Autodesk Fusion 360 part; units mm, degrees
(part 3 of 3)
sketch "Sketch2" plane through (0, 0, 6.5) normal (0, 0, 1) x (-1, 0, 0)
  line L0 (9.947362, -2.78719) -> (10.269334, 2.51736)
  arc A0 (9.726793, 3.184436) -> (10.269334, 2.51736) centre (10.86723, 3.557802) ccw
  arc A1 (9.726793, 3.184436) -> (9.129617, 4.626145) centre (0, 0) ccw
  arc A2 (9.548298, 6.176136) -> (9.129617, 4.626145) centre (10.200038, 5.168547) ccw
  line L1 (9.548298, 6.176136) -> (11.361886, 7.34922)
  spline S0 degree 5 poles (11.361886, 7.34922) (11.373267, 7.356582) (11.395716, 7.371712) (11.42845, 7.395628) (11.470315, 7.429836) (11.52024, 7.475743) (11.568461, 7.523898) (11.615662, 7.57342) (11.662318, 7.623687) (11.708575, 7.674485) (11.754381, 7.725854) (11.799563, 7.777982) (11.843926, 7.831092) (11.887356, 7.885306) (11.929863, 7.940601) (11.971521, 7.996873) (12.012444, 8.053973) (12.052738, 8.111759) (12.092468, 8.170145) (12.131644, 8.229106) (12.170248, 8.288657) (12.208248, 8.348827) (12.245612, 8.409646) (12.28233, 8.471119) (12.318409, 8.533228) (12.353869, 8.595944) (12.388733, 8.659229) (12.423021, 8.723051) (12.456745, 8.78739) (12.489908, 8.852234) (12.522508, 8.917579) (12.554541, 8.983424) (12.586002, 9.049766) (12.616893, 9.1166) (12.647217, 9.183915) (12.676977, 9.251698) (12.706181, 9.319937) (12.734832, 9.38862) (12.762935, 9.457736) (12.790491, 9.527279) (12.8175, 9.597241) (12.843962, 9.667617) (12.869878, 9.738401) (12.895248, 9.809586) (12.920074, 9.881166) (12.944358, 9.953133) (12.968101, 10.025479) (12.991304, 10.098198) (13.013969, 10.171282) (13.036098, 10.244727) (13.057689, 10.318525) (13.078745, 10.392671) (13.099265, 10.46716) (13.119249, 10.541987) (13.1387, 10.617144) (13.157616, 10.692627) (13.176, 10.768429) (13.19385, 10.844546) (13.211169, 10.920971) (13.227957, 10.997702) (13.244213, 11.074732) (13.259939, 11.152056) (13.275135, 11.229671) (13.289801, 11.307571) (13.303937, 11.385749) (13.317543, 11.464201) (13.33062, 11.54292) (13.343167, 11.621902) (13.355185, 11.701142) (13.366676, 11.780639) (13.377639, 11.860389) (13.385988, 11.924391) (13.392014, 11.972507) (13.395926, 12.004634) (13.397855, 12.02071) knots 0 0 0 0 0 0 0.01428571 0.02857143 0.04285714 0.05714286 0.07142857 0.08571429 0.1 0.11428571 0.12857143 0.14285714 0.15714286 0.17142857 0.18571429 0.2 0.21428571 0.22857143 0.24285714 0.25714286 0.27142857 0.28571429 0.3 0.31428571 0.32857143 0.34285714 0.35714286 0.37142857 0.38571429 0.4 0.41428571 0.42857143 0.44285714 0.45714286 0.47142857 0.48571429 0.5 0.51428571 0.52857143 0.54285714 0.55714286 0.57142857 0.58571429 0.6 0.61428571 0.62857143 0.64285714 0.65714286 0.67142857 0.68571429 0.7 0.71428571 0.72857143 0.74285714 0.75714286 0.77142857 0.78571429 0.8 0.81428571 0.82857143 0.84285714 0.85714286 0.87142857 0.88571429 0.9 0.91428571 0.92857143 0.94285714 0.95714286 0.97142857 0.98571429 1 1 1 1 1 1
  arc A3 (13.397855, 12.02071) -> (12.02071, 13.397855) centre (0, 0) ccw
  spline S1 degree 5 poles (12.02071, 13.397855) (12.004634, 13.395926) (11.972507, 13.392014) (11.924391, 13.385988) (11.860389, 13.377639) (11.780639, 13.366676) (11.701142, 13.355185) (11.621902, 13.343167) (11.54292, 13.33062) (11.464201, 13.317543) (11.385749, 13.303937) (11.307571, 13.289801) (11.229671, 13.275135) (11.152056, 13.259939) (11.074732, 13.244213) (10.997702, 13.227957) (10.920971, 13.211169) (10.844546, 13.19385) (10.768429, 13.176) (10.692627, 13.157616) (10.617144, 13.1387) (10.541987, 13.119249) (10.46716, 13.099265) (10.392671, 13.078745) (10.318525, 13.057689) (10.244727, 13.036098) (10.171282, 13.013969) (10.098198, 12.991304) (10.025479, 12.968101) (9.953133, 12.944358) (9.881166, 12.920074) (9.809586, 12.895248) (9.738401, 12.869878) (9.667617, 12.843962) (9.597241, 12.8175) (9.527279, 12.790491) (9.457736, 12.762935) (9.38862, 12.734832) (9.319937, 12.706181) (9.251698, 12.676977) (9.183915, 12.647217) (9.1166, 12.616893) (9.049766, 12.586002) (8.983424, 12.554541) (8.917579, 12.522508) (8.852234, 12.489908) (8.78739, 12.456745) (8.723051, 12.423021) (8.659229, 12.388733) (8.595944, 12.353869) (8.533228, 12.318409) (8.471119, 12.28233) (8.409646, 12.245612) (8.348827, 12.208248) (8.288657, 12.170248) (8.229106, 12.131644) (8.170145, 12.092468) (8.111759, 12.052738) (8.053973, 12.012444) (7.996873, 11.971521) (7.940601, 11.929863) (7.885306, 11.887356) (7.831092, 11.843926) (7.777982, 11.799563) (7.725854, 11.754381) (7.674485, 11.708575) (7.623687, 11.662318) (7.57342, 11.615662) (7.523898, 11.568461) (7.475743, 11.52024) (7.429836, 11.470315) (7.395628, 11.42845) (7.371712, 11.395716) (7.356582, 11.373267) (7.34922, 11.361886) knots -1 -1 -1 -1 -1 -1 -0.98571429 -0.97142857 -0.95714286 -0.94285714 -0.92857143 -0.91428571 -0.9 -0.88571429 -0.87142857 -0.85714286 -0.84285714 -0.82857143 -0.81428571 -0.8 -0.78571429 -0.77142857 -0.75714286 -0.74285714 -0.72857143 -0.71428571 -0.7 -0.68571429 -0.67142857 -0.65714286 -0.64285714 -0.62857143 -0.61428571 -0.6 -0.58571429 -0.57142857 -0.55714286 -0.54285714 -0.52857143 -0.51428571 -0.5 -0.48571429 -0.47142857 -0.45714286 -0.44285714 -0.42857143 -0.41428571 -0.4 -0.38571429 -0.37142857 -0.35714286 -0.34285714 -0.32857143 -0.31428571 -0.3 -0.28571429 -0.27142857 -0.25714286 -0.24285714 -0.22857143 -0.21428571 -0.2 -0.18571429 -0.17142857 -0.15714286 -0.14285714 -0.12857143 -0.11428571 -0.1 -0.08571429 -0.07142857 -0.05714286 -0.04285714 -0.02857143 -0.01428571 0 0 0 0 0 0
  line L2 (7.34922, 11.361886) -> (6.176136, 9.548298)
  arc A4 (4.626145, 9.129617) -> (6.176136, 9.548298) centre (5.168547, 10.200038) ccw
  arc A5 (4.626145, 9.129617) -> (3.184436, 9.726793) centre (0, 0) ccw
  arc A6 (3.025234, 9.791883) -> (3.184436, 9.726793) centre (3.557802, 10.86723) ccw
  line L3 (3.025234, 9.791883) -> (-3.025234, 9.791883)
  arc A7 (-3.184436, 9.726793) -> (-3.025234, 9.791883) centre (-3.557802, 10.86723) ccw
  arc A8 (-3.184436, 9.726793) -> (-4.626145, 9.129617) centre (0, 0) ccw
  arc A9 (-6.176136, 9.548298) -> (-4.626145, 9.129617) centre (-5.168547, 10.200038) ccw
  line L4 (-6.176136, 9.548298) -> (-7.34922, 11.361886)
  spline S2 degree 5 poles (-7.34922, 11.361886) (-7.356582, 11.373267) (-7.371712, 11.395716) (-7.395628, 11.42845) (-7.429836, 11.470315) (-7.475743, 11.52024) (-7.523898, 11.568461) (-7.57342, 11.615662) (-7.623687, 11.662318) (-7.674485, 11.708575) (-7.725854, 11.754381) (-7.777982, 11.799563) (-7.831092, 11.843926) (-7.885306, 11.887356) (-7.940601, 11.929863) (-7.996873, 11.971521) (-8.053973, 12.012444) (-8.111759, 12.052738) (-8.170145, 12.092468) (-8.229106, 12.131644) (-8.288657, 12.170248) (-8.348827, 12.208248) (-8.409646, 12.245612) (-8.471119, 12.28233) (-8.533228, 12.318409) (-8.595944, 12.353869) (-8.659229, 12.388733) (-8.723051, 12.423021) (-8.78739, 12.456745) (-8.852234, 12.489908) (-8.917579, 12.522508) (-8.983424, 12.554541) (-9.049766, 12.586002) (-9.1166, 12.616893) (-9.183915, 12.647217) (-9.251698, 12.676977) (-9.319937, 12.706181) (-9.38862, 12.734832) (-9.457736, 12.762935) (-9.527279, 12.790491) (-9.597241, 12.8175) (-9.667617, 12.843962) (-9.738401, 12.869878) (-9.809586, 12.895248) (-9.881166, 12.920074) (-9.953133, 12.944358) (-10.025479, 12.968101) (-10.098198, 12.991304) (-10.171282, 13.013969) (-10.244727, 13.036098) (-10.318525, 13.057689) (-10.392671, 13.078745) (-10.46716, 13.099265) (-10.541987, 13.119249) (-10.617144, 13.1387) (-10.692627, 13.157616) (-10.768429, 13.176) (-10.844546, 13.19385) (-10.920971, 13.211169) (-10.997702, 13.227957) (-11.074732, 13.244213) (-11.152056, 13.259939) (-11.229671, 13.275135) (-11.307571, 13.289801) (-11.385749, 13.303937) (-11.464201, 13.317543) (-11.54292, 13.33062) (-11.621902, 13.343167) (-11.701142, 13.355185) (-11.780639, 13.366676) (-11.860389, 13.377639) (-11.924391, 13.385988) (-11.972507, 13.392014) (-12.004634, 13.395926) (-12.02071, 13.397855) knots 0 0 0 0 0 0 0.01428571 0.02857143 0.04285714 0.05714286 0.07142857 0.08571429 0.1 0.11428571 0.12857143 0.14285714 0.15714286 0.17142857 0.18571429 0.2 0.21428571 0.22857143 0.24285714 0.25714286 0.27142857 0.28571429 0.3 0.31428571 0.32857143 0.34285714 0.35714286 0.37142857 0.38571429 0.4 0.41428571 0.42857143 0.44285714 0.45714286 0.47142857 0.48571429 0.5 0.51428571 0.52857143 0.54285714 0.55714286 0.57142857 0.58571429 0.6 0.61428571 0.62857143 0.64285714 0.65714286 0.67142857 0.68571429 0.7 0.71428571 0.72857143 0.74285714 0.75714286 0.77142857 0.78571429 0.8 0.81428571 0.82857143 0.84285714 0.85714286 0.87142857 0.88571429 0.9 0.91428571 0.92857143 0.94285714 0.95714286 0.97142857 0.98571429 1 1 1 1 1 1
  arc A10 (-12.02071, 13.397855) -> (-13.397855, 12.02071) centre (0, 0) ccw
  spline S3 degree 5 poles (-13.397855, 12.02071) (-13.395926, 12.004634) (-13.392014, 11.972507) (-13.385988, 11.924391) (-13.377639, 11.860389) (-13.366676, 11.780639) (-13.355185, 11.701142) (-13.343167, 11.621902) (-13.33062, 11.54292) (-13.317543, 11.464201) (-13.303937, 11.385749) (-13.289801, 11.307571) (-13.275135, 11.229671) (-13.259939, 11.152056) (-13.244213, 11.074732) (-13.227957, 10.997702) (-13.211169, 10.920971) (-13.19385, 10.844546) (-13.176, 10.768429) (-13.157616, 10.692627) (-13.1387, 10.617144) (-13.119249, 10.541987) (-13.099265, 10.46716) (-13.078745, 10.392671) (-13.057689, 10.318525) (-13.036098, 10.244727) (-13.013969, 10.171282) (-12.991304, 10.098198) (-12.968101, 10.025479) (-12.944358, 9.953133) (-12.920074, 9.881166) (-12.895248, 9.809586) (-12.869878, 9.738401) (-12.843962, 9.667617) (-12.8175, 9.597241) (-12.790491, 9.527279) (-12.762935, 9.457736) (-12.734832, 9.38862) (-12.706181, 9.319937) (-12.676977, 9.251698) (-12.647217, 9.183915) (-12.616893, 9.1166) (-12.586002, 9.049766) (-12.554541, 8.983424) (-12.522508, 8.917579) (-12.489908, 8.852234) (-12.456745, 8.78739) (-12.423021, 8.723051) (-12.388733, 8.659229) (-12.353869, 8.595944) (-12.318409, 8.533228) (-12.28233, 8.471119) (-12.245612, 8.409646) (-12.208248, 8.348827) (-12.170248, 8.288657) (-12.131644, 8.229106) (-12.092468, 8.170145) (-12.052738, 8.111759) (-12.012444, 8.053973) (-11.971521, 7.996873) (-11.929863, 7.940601) (-11.887356, 7.885306) (-11.843926, 7.831092) (-11.799563, 7.777982) (-11.754381, 7.725854) (-11.708575, 7.674485) (-11.662318, 7.623687) (-11.615662, 7.57342) (-11.568461, 7.523898) (-11.52024, 7.475743) (-11.470315, 7.429836) (-11.42845, 7.395628) (-11.395716, 7.371712) (-11.373267, 7.356582) (-11.361886, 7.34922) knots -1 -1 -1 -1 -1 -1 -0.98571429 -0.97142857 -0.95714286 -0.94285714 -0.92857143 -0.91428571 -0.9 -0.88571429 -0.87142857 -0.85714286 -0.84285714 -0.82857143 -0.81428571 -0.8 -0.78571429 -0.77142857 -0.75714286 -0.74285714 -0.72857143 -0.71428571 -0.7 -0.68571429 -0.67142857 -0.65714286 -0.64285714 -0.62857143 -0.61428571 -0.6 -0.58571429 -0.57142857 -0.55714286 -0.54285714 -0.52857143 -0.51428571 -0.5 -0.48571429 -0.47142857 -0.45714286 -0.44285714 -0.42857143 -0.41428571 -0.4 -0.38571429 -0.37142857 -0.35714286 -0.34285714 -0.32857143 -0.31428571 -0.3 -0.28571429 -0.27142857 -0.25714286 -0.24285714 -0.22857143 -0.21428571 -0.2 -0.18571429 -0.17142857 -0.15714286 -0.14285714 -0.12857143 -0.11428571 -0.1 -0.08571429 -0.07142857 -0.05714286 -0.04285714 -0.02857143 -0.01428571 0 0 0 0 0 0
  line L5 (-11.361886, 7.34922) -> (-9.548298, 6.176136)
  arc A11 (-9.129617, 4.626145) -> (-9.548298, 6.176136) centre (-10.200038, 5.168547) ccw
  arc A12 (-9.129617, 4.626145) -> (-9.726793, 3.184436) centre (0, 0) ccw
  arc A13 (-10.545247, 2.401806) -> (-9.726793, 3.184436) centre (-10.86723, 3.557802) ccw
  line L6 (-10.545247, 2.401806) -> (-9.854685, -2.913789)
  arc A14 (-9.726793, -3.184436) -> (-9.854685, -2.913789) centre (-10.86723, -3.557802) ccw
  arc A15 (-9.726793, -3.184436) -> (-9.129617, -4.626145) centre (0, 0) ccw
  arc A16 (-9.548298, -6.176136) -> (-9.129617, -4.626145) centre (-10.200038, -5.168547) ccw
  line L7 (-9.548298, -6.176136) -> (-11.361886, -7.34922)
  spline S4 degree 5 poles (-11.361886, -7.34922) (-11.373267, -7.356582) (-11.395716, -7.371712) (-11.42845, -7.395628) (-11.470315, -7.429836) (-11.52024, -7.475743) (-11.568461, -7.523898) (-11.615662, -7.57342) (-11.662318, -7.623687) (-11.708575, -7.674485) (-11.754381, -7.725854) (-11.799563, -7.777982) (-11.843926, -7.831092) (-11.887356, -7.885306) (-11.929863, -7.940601) (-11.971521, -7.996873) (-12.012444, -8.053973) (-12.052738, -8.111759) (-12.092468, -8.170145) (-12.131644, -8.229106) (-12.170248, -8.288657) (-12.208248, -8.348827) (-12.245612, -8.409646) (-12.28233, -8.471119) (-12.318409, -8.533228) (-12.353869, -8.595944) (-12.388733, -8.659229) (-12.423021, -8.723051) (-12.456745, -8.78739) (-12.489908, -8.852234) (-12.522508, -8.917579) (-12.554541, -8.983424) (-12.586002, -9.049766) (-12.616893, -9.1166) (-12.647217, -9.183915) (-12.676977, -9.251698) (-12.706181, -9.319937) (-12.734832, -9.38862) (-12.762935, -9.457736) (-12.790491, -9.527279) (-12.8175, -9.597241) (-12.843962, -9.667617) (-12.869878, -9.738401) (-12.895248, -9.809586) (-12.920074, -9.881166) (-12.944358, -9.953133) (-12.968101, -10.025479) (-12.991304, -10.098198) (-13.013969, -10.171282) (-13.036098, -10.244727) (-13.057689, -10.318525) (-13.078745, -10.392671) (-13.099265, -10.46716) (-13.119249, -10.541987) (-13.1387, -10.617144) (-13.157616, -10.692627) (-13.176, -10.768429) (-13.19385, -10.844546) (-13.211169, -10.920971) (-13.227957, -10.997702) (-13.244213, -11.074732) (-13.259939, -11.152056) (-13.275135, -11.229671) (-13.289801, -11.307571) (-13.303937, -11.385749) (-13.317543, -11.464201) (-13.33062, -11.54292) (-13.343167, -11.621902) (-13.355185, -11.701142) (-13.366676, -11.780639) (-13.377639, -11.860389) (-13.385988, -11.924391) (-13.392014, -11.972507) (-13.395926, -12.004634) (-13.397855, -12.02071) knots 0 0 0 0 0 0 0.01428571 0.02857143 0.04285714 0.05714286 0.07142857 0.08571429 0.1 0.11428571 0.12857143 0.14285714 0.15714286 0.17142857 0.18571429 0.2 0.21428571 0.22857143 0.24285714 0.25714286 0.27142857 0.28571429 0.3 0.31428571 0.32857143 0.34285714 0.35714286 0.37142857 0.38571429 0.4 0.41428571 0.42857143 0.44285714 0.45714286 0.47142857 0.48571429 0.5 0.51428571 0.52857143 0.54285714 0.55714286 0.57142857 0.58571429 0.6 0.61428571 0.62857143 0.64285714 0.65714286 0.67142857 0.68571429 0.7 0.71428571 0.72857143 0.74285714 0.75714286 0.77142857 0.78571429 0.8 0.81428571 0.82857143 0.84285714 0.85714286 0.87142857 0.88571429 0.9 0.91428571 0.92857143 0.94285714 0.95714286 0.97142857 0.98571429 1 1 1 1 1 1
  arc A17 (-13.397855, -12.02071) -> (-12.02071, -13.397855) centre (0, 0) ccw
  spline S5 degree 5 poles (-12.02071, -13.397855) (-12.004634, -13.395926) (-11.972507, -13.392014) (-11.924391, -13.385988) (-11.860389, -13.377639) (-11.780639, -13.366676) (-11.701142, -13.355185) (-11.621902, -13.343167) (-11.54292, -13.33062) (-11.464201, -13.317543) (-11.385749, -13.303937) (-11.307571, -13.289801) (-11.229671, -13.275135) (-11.152056, -13.259939) (-11.074732, -13.244213) (-10.997702, -13.227957) (-10.920971, -13.211169) (-10.844546, -13.19385) (-10.768429, -13.176) (-10.692627, -13.157616) (-10.617144, -13.1387) (-10.541987, -13.119249) (-10.46716, -13.099265) (-10.392671, -13.078745) (-10.318525, -13.057689) (-10.244727, -13.036098) (-10.171282, -13.013969) (-10.098198, -12.991304) (-10.025479, -12.968101) (-9.953133, -12.944358) (-9.881166, -12.920074) (-9.809586, -12.895248) (-9.738401, -12.869878) (-9.667617, -12.843962) (-9.597241, -12.8175) (-9.527279, -12.790491) (-9.457736, -12.762935) (-9.38862, -12.734832) (-9.319937, -12.706181) (-9.251698, -12.676977) (-9.183915, -12.647217) (-9.1166, -12.616893) (-9.049766, -12.586002) (-8.983424, -12.554541) (-8.917579, -12.522508) (-8.852234, -12.489908) (-8.78739, -12.456745) (-8.723051, -12.423021) (-8.659229, -12.388733) (-8.595944, -12.353869) (-8.533228, -12.318409) (-8.471119, -12.28233) (-8.409646, -12.245612) (-8.348827, -12.208248) (-8.288657, -12.170248) (-8.229106, -12.131644) (-8.170145, -12.092468) (-8.111759, -12.052738) (-8.053973, -12.012444) (-7.996873, -11.971521) (-7.940601, -11.929863) (-7.885306, -11.887356) (-7.831092, -11.843926) (-7.777982, -11.799563) (-7.725854, -11.754381) (-7.674485, -11.708575) (-7.623687, -11.662318) (-7.57342, -11.615662) (-7.523898, -11.568461) (-7.475743, -11.52024) (-7.429836, -11.470315) (-7.395628, -11.42845) (-7.371712, -11.395716) (-7.356582, -11.373267) (-7.34922, -11.361886) knots -1 -1 -1 -1 -1 -1 -0.98571429 -0.97142857 -0.95714286 -0.94285714 -0.92857143 -0.91428571 -0.9 -0.88571429 -0.87142857 -0.85714286 -0.84285714 -0.82857143 -0.81428571 -0.8 -0.78571429 -0.77142857 -0.75714286 -0.74285714 -0.72857143 -0.71428571 -0.7 -0.68571429 -0.67142857 -0.65714286 -0.64285714 -0.62857143 -0.61428571 -0.6 -0.58571429 -0.57142857 -0.55714286 -0.54285714 -0.52857143 -0.51428571 -0.5 -0.48571429 -0.47142857 -0.45714286 -0.44285714 -0.42857143 -0.41428571 -0.4 -0.38571429 -0.37142857 -0.35714286 -0.34285714 -0.32857143 -0.31428571 -0.3 -0.28571429 -0.27142857 -0.25714286 -0.24285714 -0.22857143 -0.21428571 -0.2 -0.18571429 -0.17142857 -0.15714286 -0.14285714 -0.12857143 -0.11428571 -0.1 -0.08571429 -0.07142857 -0.05714286 -0.04285714 -0.02857143 -0.01428571 0 0 0 0 0 0
  line L8 (-7.34922, -11.361886) -> (-6.176136, -9.548298)
  arc A18 (-4.626145, -9.129617) -> (-6.176136, -9.548298) centre (-5.168547, -10.200038) ccw
  arc A19 (-4.626145, -9.129617) -> (-3.184436, -9.726793) centre (0, 0) ccw
  arc A20 (-2.770942, -9.961222) -> (-3.184436, -9.726793) centre (-3.557802, -10.86723) ccw
  line L9 (-2.770942, -9.961222) -> (2.770942, -9.961222)
  arc A21 (3.184436, -9.726793) -> (2.770942, -9.961222) centre (3.557802, -10.86723) ccw
  arc A22 (3.184436, -9.726793) -> (4.626145, -9.129617) centre (0, 0) ccw
  arc A23 (6.176136, -9.548298) -> (4.626145, -9.129617) centre (5.168547, -10.200038) ccw
  line L10 (6.176136, -9.548298) -> (7.34922, -11.361886)
  spline S6 degree 5 poles (7.34922, -11.361886) (7.356582, -11.373267) (7.371712, -11.395716) (7.395628, -11.42845) (7.429836, -11.470315) (7.475743, -11.52024) (7.523898, -11.568461) (7.57342, -11.615662) (7.623687, -11.662318) (7.674485, -11.708575) (7.725854, -11.754381) (7.777982, -11.799563) (7.831092, -11.843926) (7.885306, -11.887356) (7.940601, -11.929863) (7.996873, -11.971521) (8.053973, -12.012444) (8.111759, -12.052738) (8.170145, -12.092468) (8.229106, -12.131644) (8.288657, -12.170248) (8.348827, -12.208248) (8.409646, -12.245612) (8.471119, -12.28233) (8.533228, -12.318409) (8.595944, -12.353869) (8.659229, -12.388733) (8.723051, -12.423021) (8.78739, -12.456745) (8.852234, -12.489908) (8.917579, -12.522508) (8.983424, -12.554541) (9.049766, -12.586002) (9.1166, -12.616893) (9.183915, -12.647217) (9.251698, -12.676977) (9.319937, -12.706181) (9.38862, -12.734832) (9.457736, -12.762935) (9.527279, -12.790491) (9.597241, -12.8175) (9.667617, -12.843962) (9.738401, -12.869878) (9.809586, -12.895248) (9.881166, -12.920074) (9.953133, -12.944358) (10.025479, -12.968101) (10.098198, -12.991304) (10.171282, -13.013969) (10.244727, -13.036098) (10.318525, -13.057689) (10.392671, -13.078745) (10.46716, -13.099265) (10.541987, -13.119249) (10.617144, -13.1387) (10.692627, -13.157616) (10.768429, -13.176) (10.844546, -13.19385) (10.920971, -13.211169) (10.997702, -13.227957) (11.074732, -13.244213) (11.152056, -13.259939) (11.229671, -13.275135) (11.307571, -13.289801) (11.385749, -13.303937) (11.464201, -13.317543) (11.54292, -13.33062) (11.621902, -13.343167) (11.701142, -13.355185) (11.780639, -13.366676) (11.860389, -13.377639) (11.924391, -13.385988) (11.972507, -13.392014) (12.004634, -13.395926) (12.02071, -13.397855) knots 0 0 0 0 0 0 0.01428571 0.02857143 0.04285714 0.05714286 0.07142857 0.08571429 0.1 0.11428571 0.12857143 0.14285714 0.15714286 0.17142857 0.18571429 0.2 0.21428571 0.22857143 0.24285714 0.25714286 0.27142857 0.28571429 0.3 0.31428571 0.32857143 0.34285714 0.35714286 0.37142857 0.38571429 0.4 0.41428571 0.42857143 0.44285714 0.45714286 0.47142857 0.48571429 0.5 0.51428571 0.52857143 0.54285714 0.55714286 0.57142857 0.58571429 0.6 0.61428571 0.62857143 0.64285714 0.65714286 0.67142857 0.68571429 0.7 0.71428571 0.72857143 0.74285714 0.75714286 0.77142857 0.78571429 0.8 0.81428571 0.82857143 0.84285714 0.85714286 0.87142857 0.88571429 0.9 0.91428571 0.92857143 0.94285714 0.95714286 0.97142857 0.98571429 1 1 1 1 1 1
  arc A24 (12.02071, -13.397855) -> (13.397855, -12.02071) centre (0, 0) ccw
  spline S7 degree 5 poles (13.397855, -12.02071) (13.395926, -12.004634) (13.392014, -11.972507) (13.385988, -11.924391) (13.377639, -11.860389) (13.366676, -11.780639) (13.355185, -11.701142) (13.343167, -11.621902) (13.33062, -11.54292) (13.317543, -11.464201) (13.303937, -11.385749) (13.289801, -11.307571) (13.275135, -11.229671) (13.259939, -11.152056) (13.244213, -11.074732) (13.227957, -10.997702) (13.211169, -10.920971) (13.19385, -10.844546) (13.176, -10.768429) (13.157616, -10.692627) (13.1387, -10.617144) (13.119249, -10.541987) (13.099265, -10.46716) (13.078745, -10.392671) (13.057689, -10.318525) (13.036098, -10.244727) (13.013969, -10.171282) (12.991304, -10.098198) (12.968101, -10.025479) (12.944358, -9.953133) (12.920074, -9.881166) (12.895248, -9.809586) (12.869878, -9.738401) (12.843962, -9.667617) (12.8175, -9.597241) (12.790491, -9.527279) (12.762935, -9.457736) (12.734832, -9.38862) (12.706181, -9.319937) (12.676977, -9.251698) (12.647217, -9.183915) (12.616893, -9.1166) (12.586002, -9.049766) (12.554541, -8.983424) (12.522508, -8.917579) (12.489908, -8.852234) (12.456745, -8.78739) (12.423021, -8.723051) (12.388733, -8.659229) (12.353869, -8.595944) (12.318409, -8.533228) (12.28233, -8.471119) (12.245612, -8.409646) (12.208248, -8.348827) (12.170248, -8.288657) (12.131644, -8.229106) (12.092468, -8.170145) (12.052738, -8.111759) (12.012444, -8.053973) (11.971521, -7.996873) (11.929863, -7.940601) (11.887356, -7.885306) (11.843926, -7.831092) (11.799563, -7.777982) (11.754381, -7.725854) (11.708575, -7.674485) (11.662318, -7.623687) (11.615662, -7.57342) (11.568461, -7.523898) (11.52024, -7.475743) (11.470315, -7.429836) (11.42845, -7.395628) (11.395716, -7.371712) (11.373267, -7.356582) (11.361886, -7.34922) knots -1 -1 -1 -1 -1 -1 -0.98571429 -0.97142857 -0.95714286 -0.94285714 -0.92857143 -0.91428571 -0.9 -0.88571429 -0.87142857 -0.85714286 -0.84285714 -0.82857143 -0.81428571 -0.8 -0.78571429 -0.77142857 -0.75714286 -0.74285714 -0.72857143 -0.71428571 -0.7 -0.68571429 -0.67142857 -0.65714286 -0.64285714 -0.62857143 -0.61428571 -0.6 -0.58571429 -0.57142857 -0.55714286 -0.54285714 -0.52857143 -0.51428571 -0.5 -0.48571429 -0.47142857 -0.45714286 -0.44285714 -0.42857143 -0.41428571 -0.4 -0.38571429 -0.37142857 -0.35714286 -0.34285714 -0.32857143 -0.31428571 -0.3 -0.28571429 -0.27142857 -0.25714286 -0.24285714 -0.22857143 -0.21428571 -0.2 -0.18571429 -0.17142857 -0.15714286 -0.14285714 -0.12857143 -0.11428571 -0.1 -0.08571429 -0.07142857 -0.05714286 -0.04285714 -0.02857143 -0.01428571 0 0 0 0 0 0
  line L11 (11.361886, -7.34922) -> (9.548298, -6.176136)
  arc A25 (9.129617, -4.626145) -> (9.548298, -6.176136) centre (10.200038, -5.168547) ccw
  arc A26 (9.129617, -4.626145) -> (9.726793, -3.184436) centre (0, 0) ccw
  arc A27 (9.947362, -2.78719) -> (9.726793, -3.184436) centre (10.86723, -3.557802) ccw
  circle A28 centre (0, 0) radius 1.15
  circle A29 centre (0, 0) radius 1.15
  circle A30 centre (0, 0) radius 2.25
  dimension "d19" = 4.5
  constraint concentric A1 A29
  constraint coincident A1.centre A3.centre
  measures "d19" diameter of A30
extrude "Extrude3'" add sketch "Sketch2" along normal blind 12 contours A30 picked at (1.870675, -0.168915) bodies 1 in component "Spur Gear 8 teeth"
chamfer "Chamfer1" distance 0.5 angle 45 1 faces at (0.028647, -6.971145, 0) on bodies 1 in component "Spur Gear 8 teeth"
chamfer "Chamfer2" distance 0.3 angle 45 1 faces at (0.056048, -7.275825, 6.5) on bodies 1 in component "Spur Gear 8 teeth"
chamfer "Chamfer3" distance 0.2 angle 45 1 faces at (-1.870675, 0.168915, 18.5) on bodies 1 in component "Spur Gear 8 teeth"
component "Spur Gear 8 teeth (1)" placed x (1, 0, 0) y (0, 1, 0) z (0, 0, 1) at (0, 0, 0)
component "Spur Gear 8 teeth" placed x (1, 0, 0) y (0, 1, 0) z (0, 0, 1) at (0, 0, 0)

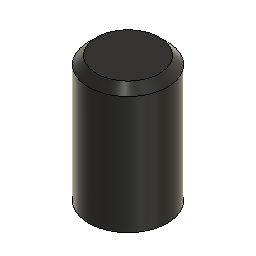
design "Pin"
part number: 2026-05-27-02-31-01-321
Autodesk Fusion 360 part; units mm, degrees
sketch "Sketch1" plane through (0, 0, 0) normal (0, 0, 1) x (1, 0, 0)
  circle A0 centre (40, 25) radius 2.5
  dimension "d1" = 5
  measures "d1" diameter of A0
extrude "Extrude1" add sketch "Sketch1" along normal blind 8
chamfer "Chamfer1" distance 0.5 angle 45 1 edges at (37.6692, 24.096, 8)

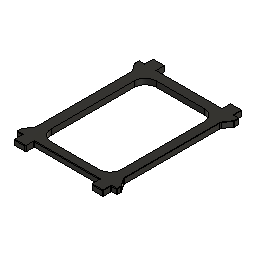
design "Rama fata-spate"
part number: 2026-05-26-13-04-27-356
Autodesk Fusion 360 part; units mm, degrees
sketch "Sketch1" plane through (0, 0, 0) normal (0, 0, 1) x (1, 0, 0)
  line L0 (-23, 48.647989) -> (-57, 48.647989)
  line L1 (-65, 56.647989) -> (-65, 115.647989)
  line L2 (-15, 56.647989) -> (-15, 115.647989)
  line L3 (-23, 123.647989) -> (-57, 123.647989)
  arc A0 (-65, 56.647989) -> (-57, 48.647989) centre (-57, 56.647989) ccw
  arc A1 (-57, 123.647989) -> (-65, 115.647989) centre (-57, 115.647989) ccw
  arc A2 (-23, 48.647989) -> (-15, 56.647989) centre (-23, 56.647989) ccw
  arc A3 (-15, 115.647989) -> (-23, 123.647989) centre (-23, 115.647989) ccw
  line L4 (-16.7, 43.000001) -> (-16.7, 37.000001)
  line L5 (-16.7, 37.000001) -> (-8.7, 37.000001)
  line L6 (-8.7, 37.000001) -> (-8.7, 43.000001)
  line L7 (-8.7, 43.000001) -> (-4.7, 43.000001)
  line L8 (-4.7, 43.000001) -> (-4.7, 45.984132)
  line L9 (-16.7, 43.000001) -> (-63.7, 43.000001)
  line L10 (-63.7, 43.000001) -> (-63.7, 37.000001)
  line L11 (-63.7, 37.000001) -> (-71.7, 37.000001)
  line L12 (-71.7, 37.000001) -> (-71.7, 43.000001)
  line L13 (-71.7, 43.000001) -> (-75.7, 43.000001)
  line L14 (-75.7, 43.000001) -> (-75.7, 45.984132)
  line L15 (-8.7, 52.631739) -> (-8.7, 120.368262)
  line L16 (-4.7, 127.01587) -> (-4.7, 130.000001)
  line L17 (-4.7, 130.000001) -> (-8.7, 130.000001)
  line L18 (-8.7, 130.000001) -> (-8.7, 136.000001)
  line L19 (-8.7, 136.000001) -> (-16.7, 136.000001)
  line L20 (-16.7, 136.000001) -> (-16.7, 130.000001)
  line L21 (-71.7, 52.631739) -> (-71.7, 120.368263)
  line L22 (-75.7, 127.01587) -> (-75.7, 130.000001)
  line L23 (-75.7, 130.000001) -> (-71.7, 130.000001)
  line L24 (-71.7, 130.000001) -> (-71.7, 136.000001)
  line L25 (-71.7, 136.000001) -> (-63.7, 136.000001)
  line L26 (-63.7, 136.000001) -> (-63.7, 130.000002)
  line L27 (-63.7, 130.000002) -> (-16.7, 130.000001)
  line L28 (-75.518557, 46.558557) -> (-72.062887, 51.482887)
  line L29 (-75.518557, 126.441444) -> (-72.062887, 121.517114)
  line L30 (-4.881443, 126.441444) -> (-8.337113, 121.517114)
  line L31 (-4.881443, 46.558557) -> (-8.337113, 51.482887)
  arc A4 (-75.518557, 46.558557) -> (-75.7, 45.984132) centre (-74.7, 45.984132) ccw
  arc A5 (-72.062887, 51.482887) -> (-71.7, 52.631739) centre (-73.7, 52.631739) ccw
  arc A6 (-71.7, 120.368263) -> (-72.062887, 121.517114) centre (-73.7, 120.368263) ccw
  arc A7 (-75.7, 127.01587) -> (-75.518557, 126.441444) centre (-74.7, 127.01587) ccw
  arc A8 (-4.881443, 126.441444) -> (-4.7, 127.01587) centre (-5.7, 127.01587) ccw
  arc A9 (-8.337113, 121.517114) -> (-8.7, 120.368262) centre (-6.7, 120.368262) ccw
  arc A10 (-4.7, 45.984132) -> (-4.881443, 46.558557) centre (-5.7, 45.984132) ccw
  arc A11 (-8.7, 52.631739) -> (-8.337113, 51.482887) centre (-6.7, 52.631739) ccw
  point P0 (-15, 48.647989)
  point P1 (-65, 48.647989)
  point P2 (-65, 123.647989)
  point P3 (-8.7, 52.000001)
  point P4 (-71.7, 52.000001)
  point P5 (-8.7, 121.000001)
  point P6 (-71.7, 121.000001)
  dimension "d1" = 50
  dimension "d2" = 75
  dimension "d3" = 8
  dimension "d4" = 8
  dimension "d5" = 8
  dimension "d6" = 8
  dimension "d8" = 8
  dimension "d9" = 6
  dimension "d10" = 4
  dimension "d20" = 47
  dimension "d21" = 6
  dimension "d22" = 8
  dimension "d23" = 6
  dimension "d24" = 4
  dimension "d28" = 69
  dimension "d31" = 4
  dimension "d32" = 6
  dimension "d33" = 8
  dimension "d34" = 6
  dimension "d35" = 69
  dimension "d38" = 4
  dimension "d39" = 6
  dimension "d40" = 8
  dimension "d45" = 1
  dimension "d46" = 2
  dimension "d47" = 2
  dimension "d48" = 1
  dimension "d49" = 1
  dimension "d50" = 2
  dimension "d51" = 1
  dimension "d52" = 2
  constraint horizontal L0
  constraint perpendicular L0 L1
  constraint perpendicular L0 L2
  constraint perpendicular L1 L3
  constraint tangent L1 A0
  constraint tangent L0 A0
  constraint tangent L1 A1
  constraint tangent L3 A1
  constraint tangent L0 A2
  constraint tangent L2 A2
  constraint tangent L3 A3
  constraint tangent L2 A3
  constraint perpendicular L4 L5
  constraint perpendicular L5 L6
  constraint perpendicular L6 L7
  constraint perpendicular L7 L8
  constraint perpendicular L4 L9
  constraint perpendicular L9 L10
  constraint perpendicular L10 L11
  constraint perpendicular L11 L12
  constraint perpendicular L12 L13
  constraint perpendicular L13 L14
  constraint perpendicular L16 L17
  constraint perpendicular L17 L18
  constraint perpendicular L18 L19
  constraint perpendicular L19 L20
  constraint perpendicular L22 L23
  constraint perpendicular L23 L24
  constraint perpendicular L24 L25
  constraint perpendicular L25 L26
  constraint tangent L14 A4
  constraint tangent L28 A4
  constraint tangent L28 A5
  constraint tangent L21 A5
  constraint tangent L21 A6
  constraint tangent L29 A6
  constraint tangent L29 A7
  constraint tangent L22 A7
  constraint tangent L30 A8
  constraint tangent L16 A8
  constraint tangent L15 A9
  constraint tangent L30 A9
  constraint tangent L8 A10
  constraint tangent L31 A10
  constraint tangent L31 A11
  constraint tangent L15 A11
  measures "d3" radius of A0
  measures "d4" radius of A1
  measures "d5" radius of A2
  measures "d6" radius of A3
  measures "d45" radius of A4
  measures "d46" radius of A5
  measures "d47" radius of A6
  measures "d48" radius of A7
  measures "d49" radius of A8
  measures "d50" radius of A9
  measures "d51" radius of A10
  measures "d52" radius of A11
extrude "Extrude1" add sketch "Sketch1" along normal blind 4 contours L4 L5 L6 L7 L8 L9 L10 L11 L12 L13 L14 L15 L16 L17 L18 L19 L20 L21 L22 L23 L24 L25 L26 L27 L28 L29 L30 L31 A4 A5 A6 A7 A8 A9 A10 A11 picked at (-69.466667, 96.215997)
chamfer "Chamfer1" distance 0.4 angle 45 5 faces at (-66.366667, 37.000001, 1.333333) (-14.033333, 37.000001, 1.333333) (-73.033333, 43.000001, 1.333333) (-32.366667, 43.000001, 1.333333) (-7.366667, 43.000001, 1.333333)
chamfer "Chamfer2" distance 0.2 angle 45 11 faces at (-8.7, 39.133334, 1.6) (-8.7, 75.21058, 1.333333) (-8.673433, 120.693164, 2.666667) (-6.033333, 124.800001, 1.333333) (-4.700832, 126.975087, 2.666667) (-4.7, 128.01058, 1.333333) (-8.594439, 51.990567, 2.666667) (-6.033333, 48.200001, 1.333333) (-4.799001, 46.417952, 2.666667) (-4.7, 44.261378, 1.333333) (-8.7, 132.000001, 1.333333)
chamfer "Chamfer3" distance 0.1 angle 45 5 faces at (-6.1, 130.000001, 1.466667) (-48.033333, 130.000001, 1.333333) (-11.5, 136.000001, 1.333333) (-69.033333, 136.000001, 1.333333) (-74.366667, 130.000001, 1.333333)
